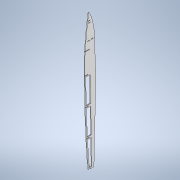
# Autodesk Inventor part: stringer
Saved by Autodesk Inventor 2022 (Build 260153000, 153)
## iProperties
Created: 2021-04-24
Part Number: stringer
Material: Generic
Document SubType Name: Modeling
Designer: kardo
Density: 1 g/cm^3
Appearance: Default
Mass: 50.4716 g
Surface Area: 402.116 cm^2
Volume: 50.4716 cm^3
Author: kardo
Autodesk Inventor part; units mm, degrees
ref_plane "YZ Plane" through (0, 0, 0) normal (1, 0, 0) x (0, 1, 0)
ref_plane "XZ Plane" through (0, 0, 0) normal (0, 1, 0) x (-1, 0, 0)
ref_plane "XY Plane" through (0, 0, 0) normal (0, 0, 1) x (1, 0, 0)
derived "frame_outline.ipt"
sketch "stringer" plane through (81, 0, 0) normal (1, 0, 0) x (0, 1, 0)
  line L0 (0, 0) -> (130.35, 9.115)
  line L1 (0, 4.352) -> (-363, 13.6)
  line L2 (-363, 18.496) -> (-297.6664, 19.4083)
  line L3 (-37.9005, 25.6108) -> (-277.6703, 19.7906)
  line L4 (28.4595, 27.2216) -> (-37.9005, 25.6108)
  line L5 (94.8, 28.832) -> (28.4595, 27.2216)
  line L6 (130.2942, 9.913) -> (0, 0.802)
  line L7 (-363, 37.2757) -> (-363, 13.6)
  line L8 (-366.2705, 37.7415) -> (-363, 38.08) construction
  line L9 (-362.9176, 37.2843) -> (-363, 37.2757)
  line L10 (0, 0.802) -> (0, 4.352)
  line L11 (0, 86.9585) -> (0, -19.4928) construction
  line L12 (-242, 86.9585) -> (-242, -19.4928) construction
  line L13 (-121, 86.9585) -> (-121, -19.4928) construction
  line L14 (94.8, 86.9585) -> (94.8, -19.4928) construction
  line L15 (133.5641, -36.8495) -> (121.9065, 129.8631) construction
  spline S0 degree 4 poles (0, 54.4) (23.3745, 54.808) (84.9613, 55.883) (149.0088, 47.5461) (201.9993, 42.6196) (237, 36.448) knots 0 0 0 0 0 0.379537 1 1 1 1 1
  spline S1 degree 3 poles (130.35, 9.115) (172.0992, 12.0344) (220.2053, 21.9532) (237, 36.448) knots 0 0 0 0 1 1 1 1
  spline S2 degree 3 poles (-363, 38.08) (-277.2033, 46.9603) (-131.9759, 52.0964) (0, 54.4) knots 0 0 0 0 1 1 1 1
  spline S3 degree 3 poles (-297.6664, 19.4083) (-291.0004, 19.5014) (-284.3349, 19.6288) (-277.6703, 19.7906) knots 0 0 0 0 1 1 1 1
  spline S4 degree 3 poles (235.1399, 35.9612) (233.6795, 34.8294) (230.3506, 32.6128) (225.2739, 29.9832) (219.5898, 27.4703) (214.5879, 25.5567) (207.8452, 23.2931) (202.0896, 21.5874) (194.5202, 19.5924) (188.1953, 18.1084) (180.0289, 16.3987) (173.318, 15.1493) (164.7832, 13.7404) (157.8689, 12.7377) (149.1938, 11.6447) (140.5245, 10.7146) (133.6763, 10.1495) (130.2942, 9.913) knots 0 0 0 0 0.081171 0.162342 0.202927 0.284098 0.324683 0.405854 0.446439 0.52761 0.568196 0.649366 0.689952 0.771123 0.811708 0.892879 0.97405 0.97405 0.97405 0.97405
  spline S5 degree 3 poles (0.014, 53.6001) (-21.9803, 53.2162) (-61.1142, 52.4067) (-105.9489, 51.1914) (-139.2434, 50.1509) (-161.2109, 49.3919) (-188.2265, 48.3595) (-209.4207, 47.4659) (-235.2328, 46.2623) (-255.275, 45.2293) (-279.4102, 43.8486) (-297.9213, 42.6717) (-319.9057, 41.108) (-340.6567, 39.451) (-355.773, 38.0238) (-362.9176, 37.2843) knots 0 0 0 0 0.166667 0.291667 0.333333 0.416667 0.458333 0.541667 0.583333 0.666667 0.708333 0.791667 0.833333 0.916667 1 1 1 1
  spline S6 degree 3 poles (0.014, 53.6001) (3.4093, 53.6594) (10.1989, 53.7777) (18.6916, 53.8929) (27.1921, 53.964) (33.9997, 53.9789) (42.5184, 53.932) (49.3401, 53.8379) (57.8725, 53.6429) (64.7007, 53.4237) (73.2321, 53.0704) (80.0508, 52.7255) (88.556, 52.2228) (95.3407, 51.7673) (103.7841, 51.1437) (110.5031, 50.6066) (118.8467, 49.8982) (125.4741, 49.3055) (133.6924, 48.5392) (140.2125, 47.9083) (148.2924, 47.1014) (154.7, 46.442) (162.6413, 45.6014) (168.9413, 44.9154) (176.7565, 44.0383) (182.9642, 43.3193) (190.6787, 42.393) (196.8193, 41.6268) (206.0017, 40.4288) (218.2121, 38.7331) (228.9412, 37.0365) (235.1399, 35.9612) knots 0 0 0 0 0.041348 0.082696 0.10337 0.144718 0.165392 0.20674 0.227414 0.268763 0.289437 0.330785 0.351459 0.392807 0.413481 0.454829 0.475503 0.516851 0.537525 0.578873 0.599547 0.640895 0.661569 0.702917 0.723591 0.764939 0.785613 0.826962 0.847636 0.909658 0.992354 0.992354 0.992354 0.992354
  spline S7 degree 2 poles (0, 55.974) (-217.9618, 52.7695) (-363, 39.654) knots 0 0 0 1 1 1
  line L16 (128.6952, 32.7794) -> (236.1697, 36.5325) construction
  line L17 (129.046, 27.7634) -> (235.7442, 35.2245) construction
  line L18 (130.1045, 12.6264) -> (128.1076, 12.5117) construction
  line L19 (0, 5.1533) -> (0, 4.352)
  line L20 (128.2991, 9.7735) -> (128.1076, 12.5117)
  line L21 (128.1076, 12.5117) -> (0, 5.1533)
  point P0 (94.8, 33.184)
  point P1 (0, 40.4654)
  point P2 (-121, 37.5562)
  point P3 (-242, 33.6806)
  point P4 (-363, 28.288)
  point P5 (128.0674, 41.7579)
  point P6 (128.638, 33.5972)
  point P7 (129.2087, 25.4364)
  point P8 (129.7793, 17.2757)
  point P9 (196.0258, 32.4471)
  point P10 (203.9273, 35.4065)
  point P11 (195.677, 37.4349)
  point P12 (196.2351, 29.4544)
  point P13 (204.1018, 30.4096)
  point P14 (203.8226, 38.4047)
extrude "Extrusion1" add sketch "stringer" along normal blind 3 contours L1 L7 L9 S5 S6 S4 L6 L20 L21 L19
sketch "Sketch2" plane through (81, -363, 13.6) normal (-1, 0, 0) x (0, 0, 1)
  spline S0 degree 2 poles (42.374, 363) (39.1695, 145.0382) (26.054, 0) knots 0 0 0 1 1 1 projected
  line L0 (12.0108, 325.0995) -> (6.1906, 85.3297) projected
  line L1 (13.6216, 391.4595) -> (12.0108, 325.0995) projected
  line L2 (15.232, 457.8) -> (13.6216, 391.4595) projected
  spline S1 degree 3 poles (5.8083, 65.3336) (5.9014, 71.9996) (6.0288, 78.6651) (6.1906, 85.3297) knots 0 0 0 0 1 1 1 1 projected
  line L3 (4.896, 0) -> (5.8083, 65.3336) projected
  line L4 (73.3585, 457.8) -> (-33.0928, 457.8) construction
  line L5 (73.3585, 363) -> (-33.0928, 363) construction
  line L6 (73.3585, 242) -> (-33.0928, 242) construction
  line L7 (73.3585, 121) -> (-33.0928, 121) construction
  line L8 (23.6757, 0) -> (0, 0) projected
  line L9 (40.8, 363) -> (26.8654, 363)
  line L10 (26.8654, 363) -> (26.8654, 365)
  line L11 (26.8654, 365) -> (40.8349, 365)
  line L12 (9.9936, 242) -> (39.6598, 242)
  line L13 (23.9562, 242) -> (23.9562, 244)
  line L14 (23.9562, 244) -> (39.7214, 244)
  line L15 (7.0564, 121) -> (34.6037, 121)
  line L16 (20.0806, 121) -> (20.0806, 123)
  line L17 (20.0806, 123) -> (34.7113, 123)
  line L18 (4.896, 0) -> (26.054, 0)
  line L19 (23.6757, 0) -> (0, 0) projected
  line L20 (14.688, 0) -> (14.688, 2)
  line L21 (14.688, 2) -> (26.2341, 2)
  line L22 (15.232, 457.8) -> (38.9981, 457.8)
  spline S2 degree 4 poles (40.8, 363) (41.208, 386.3745) (42.283, 447.9613) (33.9461, 512.0088) (29.0196, 564.9993) (22.848, 600) knots 0 0 0 0 0 0.379537 1 1 1 1 1 projected
  line L23 (19.584, 457.8) -> (19.584, 455.8)
  line L24 (19.584, 455.8) -> (39.1354, 455.8)
  line L25 (26.8654, 363) -> (12.9308, 363)
  line L26 (3.6757, 492.7793) -> (11.8364, 492.2087)
  line L27 (11.8364, 492.2087) -> (11.6969, 490.2136)
  line L28 (11.6969, 490.2136) -> (3.5362, 490.7842)
  line L29 (3.5362, 490.7842) -> (3.6757, 492.7793)
  line L30 (19.9972, 491.638) -> (28.1579, 491.0674)
  line L31 (28.1579, 491.0674) -> (28.0184, 489.0723)
  line L32 (28.0184, 489.0723) -> (19.8577, 489.6429)
  line L33 (19.8577, 489.6429) -> (19.9972, 491.638)
  point P0 (-13.6, 363)
  point P1 (11.9487, 0)
  dimension "d3" = 2
  dimension "d6" = 2
  dimension "d9" = 2
  dimension "d12" = 2
  dimension "d15" = 2
  dimension "d33" = 2
  constraints: 48 end point, 19 point on line, 5 horizontal, 5 vertical, 4 perpendicular, 3 parallel, 1 collinear, 8 other
  measures "d3" distance between parallel lines of L9 L11
  measures "d6" distance between parallel lines of L6 L14
  measures "d9" distance between parallel lines of L7 L17
  measures "d12" distance between parallel lines of L8 L21
  measures "d15" distance between parallel lines of L22 L24
  measures "d33" distance of L30.end L31.end
extrude "Extrusion2" cut sketch "Sketch2" against normal through all contours S0 L12 L13 L14 | S0 L15 L16 L17 | S0 L18 L8 L20 L21 | L10 L11 S2 L9 | L22 S2 L24 L23 | L26 L27 L28 L29 | L30 L31 L32 L33
sketch "Sketch3" plane through (81, -363, 13.6) normal (-1, 0, 0) x (0, 0, 1)
  line L0 (13.6216, 391.4595) -> (12.0108, 325.0995) projected
  line L1 (12.0108, 325.0995) -> (6.1906, 85.3297) projected
  spline S0 degree 3 poles (5.8083, 65.3336) (5.9014, 71.9996) (6.0288, 78.6651) (6.1906, 85.3297) knots 0 0 0 0 1 1 1 1 projected
  line L2 (4.896, 0) -> (5.8083, 65.3336) projected
  line L3 (39.9999, 363) -> (26.8654, 363) projected
  line L4 (23.9562, 244) -> (37.1795, 244) projected
  line L5 (37.1184, 242) -> (23.9562, 242) projected
  line L6 (20.0806, 123) -> (32.405, 123) projected
  line L7 (32.3037, 121) -> (20.0806, 121) projected
  line L8 (14.688, 2) -> (23.8811, 2) projected
  line L9 (35.9293, 359) -> (16.8337, 359)
  line L10 (16.8337, 359) -> (14.1393, 248)
  line L11 (14.1393, 248) -> (33.3004, 248)
  line L12 (33.3004, 248) -> (35.9293, 359)
  line L13 (32.9945, 238) -> (13.8965, 238)
  line L14 (13.8965, 238) -> (11.2021, 127)
  line L15 (11.2021, 127) -> (28.6049, 127)
  line L16 (28.6049, 127) -> (32.9945, 238)
  line L17 (28.0984, 117) -> (10.9594, 117)
  line L18 (10.9594, 117) -> (8.9798, 6)
  line L19 (8.9798, 6) -> (20.2816, 6)
  line L20 (20.2816, 6) -> (28.0984, 117)
  line L21 (35.9293, 359) -> (39.9293, 359) construction
  line L22 (33.3004, 248) -> (37.3004, 248) construction
  line L23 (32.9945, 238) -> (36.9945, 238) construction
  line L24 (28.6049, 127) -> (32.6049, 127) construction
  line L25 (28.0984, 117) -> (32.0984, 117) construction
  line L26 (24.2816, 6) -> (20.2816, 6) construction
  line L27 (12.8337, 359) -> (16.8337, 359) construction
  line L28 (14.1393, 248) -> (10.1393, 248) construction
  line L29 (13.8965, 238) -> (9.8965, 238) construction
  line L30 (11.2021, 127) -> (7.2021, 127) construction
  line L31 (10.9594, 117) -> (6.9594, 117) construction
  line L32 (8.9798, 6) -> (4.9798, 6) construction
  point P0 (-13.6, 363)
  dimension "d23" = 4
  dimension "d24" = 4
  dimension "d25" = 4
  dimension "d26" = 4
  dimension "d27" = 4
  dimension "d28" = 4
  dimension "d29" = 4
  constraints: 49 end point, 12 collinear, 11 equal length, 6 parallel, 6 point on line, 9 other
  measures "d23" distance of L9.start L21.end
  measures "d24" distance between parallel lines of L7 L17
  measures "d25" distance between parallel lines of L6 L15
  measures "d26" distance between parallel lines of L8 L19
  measures "d27" distance between parallel lines of L5 L13
  measures "d28" distance between parallel lines of L4 L11
  measures "d29" distance between parallel lines of L3 L9
extrude "Extrusion3" cut sketch "Sketch3" against normal through all
sketch "Sketch4" plane through (81, -363, 13.6) normal (-1, 0, 0) x (0, 0, 1)
  line L0 (19.1794, 491.6952) -> (22.9325, 599.1697) construction
  line L1 (14.1634, 492.046) -> (21.6245, 598.7442) construction
  line L2 (15.8544, 559.2351) -> (23.8349, 558.677)
  line L3 (23.8349, 558.677) -> (23.6954, 556.6819)
  line L4 (23.6954, 556.6819) -> (15.7149, 557.2399)
  line L5 (15.7149, 557.2399) -> (15.8544, 559.2351)
  line L6 (16.8096, 567.1018) -> (24.8047, 566.8226)
  line L7 (24.8047, 566.8226) -> (24.7349, 564.8239)
  line L8 (24.7349, 564.8239) -> (16.7398, 565.103)
  line L9 (16.7398, 565.103) -> (16.8096, 567.1018)
  point P0 (-13.6, 363)
  point P1 (18.8471, 559.0258)
  point P2 (21.8065, 566.9273)
  dimension "d40" = 2
  dimension "d41" = 2
  constraints: 16 end point, 4 parallel, 2 coincident, 2 perpendicular
  measures "d40" distance of L2.end L3.end
  measures "d41" distance of L6.end L7.end
extrude "Extrusion4" cut sketch "Sketch4" against normal through all
fillet "Fillet1" radius 1.3333 12 edges at (82.5, -115, 27.7393) (82.5, -236, 24.8021) (82.5, -357, 22.5798) (82.5, -357, 33.8816) (82.5, -236, 42.2049) (82.5, -115, 46.9004) (82.5, -4, 30.4337) (82.5, -125, 27.4965) (82.5, -246, 24.5594) (82.5, -246, 41.6984) (82.5, -125, 46.5945) (82.5, -4, 49.5293)
equation "\"d1\" = stringer_thickness"
equation "\"d3\" = bulkhead_thickness"
equation "\"d6\" = bulkhead_thickness"
equation "\"d9\" = bulkhead_thickness"
equation "\"d12\" = bulkhead_thickness"
equation "\"d15\" = bulkhead_thickness"
equation "\"d33\" = bulkhead_thickness"
equation "\"d23\" = inset"
equation "\"d24\" = inset"
equation "\"d25\" = inset"
equation "\"d26\" = inset"
equation "\"d27\" = inset"
equation "\"d28\" = inset"
equation "\"d29\" = inset"
equation "\"d40\" = bulkhead_thickness"
equation "\"d41\" = bulkhead_thickness"
equation "\"d32\" = 0.333333 * inset"
equation "\"stringer_thickness\" = 3"
equation "\"bulkhead_thickness\" = 2"
equation "\"inset\" = 4"
body "Solid1"
